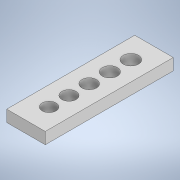
# Autodesk Inventor part: Test Block for Inserts
Saved by Autodesk Inventor 2021 (Build 250183000, 183)
## iProperties
Created: 2021-08-02
Part Number: Test Block for Inserts
Material: Generic
Document SubType Name: Modeling
Designer: cmzgt
Density: 1 g/cm^3
Appearance: Default
Author: cmzgt
Autodesk Inventor part; units mm, degrees
ref_plane "YZ Plane" through (0, 0, 0) normal (1, 0, 0) x (0, 1, 0)
ref_plane "XZ Plane" through (0, 0, 0) normal (0, 1, 0) x (-1, 0, 0)
ref_plane "XY Plane" through (0, 0, 0) normal (0, 0, 1) x (1, 0, 0)
sketch "Sketch1" plane through (0, 0, 0) normal (0, 1, 0) x (-1, 0, 0)
  line L0 (-5, -21.8883) -> (5, -21.8883)
  line L1 (5, -21.8883) -> (5, 11.3117)
  line L2 (5, 11.3117) -> (-5, 11.3117)
  line L3 (-5, 11.3117) -> (-5, -21.8883)
  circle A0 centre (0, 0.1617) radius 1.85
  circle A1 centre (0, -5.0883) radius 1.9
  line L4 (0, 11.3117) -> (0, -21.8883) construction
  circle A2 centre (0, 5.3117) radius 1.8
  circle A3 centre (0, -10.4383) radius 1.95
  circle A4 centre (0, -15.8883) radius 2
  dimension "d1" = 10
  dimension "d2" = 3.7
  dimension "d3" = 3.8
  dimension "d4" = 1.5
  dimension "d5" = 3.6
  dimension "d6" = 1.5
  dimension "d8" = 3.9
  dimension "d9" = 1.5
  dimension "d10" = 4
  dimension "d11" = 1.5
  dimension "d12" = 6
  dimension "d13" = 6
  constraints: 10 end point, 5 centre point, 4 point on line, 2 midpoint, 2 parallel, 1 horizontal, 1 perpendicular
  measures "d1" distance of L1.end L2.end
  measures "d2" diameter of A0
  measures "d3" diameter of A1
  measures "d5" diameter of A2
  measures "d8" diameter of A3
  measures "d10" diameter of A4
  measures "d12" distance from line of L0 A4.centre
  measures "d13" distance from line of L2 A2.centre
extrude "Extrusion1" add sketch "Sketch1" along normal blind 3
body "Solid1"
